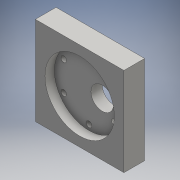
# Autodesk Inventor part: motorHolder57mm
Saved by Autodesk Inventor 2016 (Build 200138000, 138)
## iProperties
Created: 2016-05-09
Part Number: motorHolder57mm
Material: Generic
Document SubType Name: Modeling
Designer: hesaon
Density: 1 g/cm^3
Appearance: Default
Author: hesaon
Autodesk Inventor part; units mm, degrees
ref_plane "YZ Plane" through (0, 0, 0) normal (1, 0, 0) x (0, 1, 0)
ref_plane "XZ Plane" through (0, 0, 0) normal (0, 1, 0) x (-1, 0, 0)
ref_plane "XY Plane" through (0, 0, 0) normal (0, 0, 1) x (1, 0, 0)
sketch "Sketch1" plane through (0, 0, 0) normal (0, 1, 0) x (-1, 0, 0)
  line L0 (0, 0) -> (47, 0)
  line L1 (47, 0) -> (47, -47)
  line L2 (47, -47) -> (0, -47)
  line L3 (0, -47) -> (0, 0)
  circle A0 centre (23.5, -23.5) radius 18.4
  dimension "width" = 47
  dimension "height" = 47
  dimension "d2" = 36.8
  dimension "d3" = 23.5
  dimension "d4" = 23.5
  constraints: 8 end point, 2 parallel, 1 centre point, 1 horizontal, 1 perpendicular
  measures "width" distance of L1.end L2.end
  measures "height" distance of L0.end L1.end
  measures "d2" diameter of A0
  measures "d3" distance from line of L0 A0.centre
  measures "d4" distance from line of L3 A0.centre
extrude "Extrusion1" add sketch "Sketch1" along normal blind 5
sketch "Sketch2" plane through (0, 5, 0) normal (0, 1, 0) x (1, 0, 0)
  line L0 (-47, 0) -> (0, 0) projected
  line L1 (0, 47) -> (-47, 47) projected
  line L2 (0, 0) -> (-47, 0)
  line L3 (-47, 0) -> (-47, 47)
  line L4 (-47, 47) -> (0, 47)
  line L5 (0, 47) -> (0, 0)
  circle A0 centre (-23.5, 8) radius 1.5
  line L6 (-47, 47) -> (-47, 0) projected
  line L7 (0, 0) -> (0, 47) projected
  circle A1 centre (-10.0766, 15.75) radius 1.5
  circle A2 centre (-10.0766, 31.25) radius 1.5
  circle A3 centre (-23.5, 39) radius 1.5
  circle A4 centre (-36.9234, 31.25) radius 1.5
  circle A5 centre (-36.9234, 15.75) radius 1.5
  circle A6 centre (-16.5, 23.5) radius 6
  point P0 (-23.5, 23.5)
  dimension "d10" = 3
  dimension "d11" = 23.5
  dimension "d13" = 15.5
  dimension "d16" = 360
  dimension "d18" = 12
  dimension "d19" = 7
  dimension "d20" = 23.5
  dimension "d21" = 23.5
  dimension "d22" = 23.5
  constraints: 8 end point, 7 centre point, 2 parallel, 1 horizontal, 1 perpendicular, 13 other
  measures "d10" diameter of A0
  measures "d11" distance from line of L5 A0.centre
  measures "d13" distance of point (-23.5, 23.5) A0.centre
  measures "d18" diameter of A6
  measures "d19" distance of A6.centre point (-23.5, 23.5)
  measures "d20" distance from line of L1 A6.centre
  measures "d21" distance from line of L3 point (-23.5, 23.5)
  measures "d22" distance from line of L1 point (-23.5, 23.5)
extrude "Extrusion2" add sketch "Sketch2" along normal blind 6
equation "\"d3\" = 0.5 * height"
equation "\"d4\" = 0.5 * width"
equation "\"d11\" = 0.5 * height"
body "Solid1"
